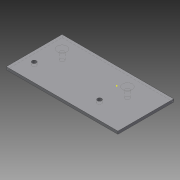
# Autodesk Inventor part: Power circuit support surface
Saved by Autodesk Inventor 2015 (Build 190159000, 159)
## iProperties
Created: 2019-05-03
Part Number: Power circuit support surface
Material: Generic
Document SubType Name: Modeling
Designer: Toby
Density: 1 g/cm^3
Appearance: Default
Author: Toby
Autodesk Inventor part; units mm, degrees
ref_plane "YZ Plane" through (0, 0, 0) normal (1, 0, 0) x (0, 1, 0)
ref_plane "XZ Plane" through (0, 0, 0) normal (0, 1, 0) x (-1, 0, 0)
ref_plane "XY Plane" through (0, 0, 0) normal (0, 0, 1) x (1, 0, 0)
sketch "Sketch1" plane through (0, 0, 0) normal (0, 0, 1) x (1, 0, 0)
  line L0 (-51.5762, 12.5065) -> (28.4238, 12.5065)
  line L1 (28.4238, 12.5065) -> (28.4238, -27.4935)
  line L2 (28.4238, -27.4935) -> (-51.5762, -27.4935)
  line L3 (-51.5762, -27.4935) -> (-51.5762, 12.5065)
  point P0 (0, 0)
  dimension "d0" = 80
  dimension "d1" = 40
  constraints: 8 end point, 2 parallel, 1 horizontal, 1 perpendicular
  measures "d0" distance between parallel lines of L1 L3
  measures "d1" distance of L2.end L0.start
extrude "Extrusion1" add sketch "Sketch1" along normal blind 2
sketch "Sketch2" plane through (0, 0, 2) normal (0, 0, 1) x (1, 0, 0)
  line L0 (-51.5762, 12.5065) -> (-51.5762, -27.4935) projected
  line L1 (-51.5762, -27.4935) -> (28.4238, -27.4935) projected
  point P0 (0, 0)
  point P1 (-44.5762, -14.4935)
  point P2 (2.2739, -14.4935)
  dimension "d4" = 46.8502
  dimension "d5" = 7
  dimension "d6" = 13
  dimension "d7" = 13
  measures "d4" distance of point (2.274, -14.494) point (-44.576, -14.494)
  measures "d5" distance from line of L0 point (-44.576, -14.494)
  measures "d6" distance from line of L1 point (-44.576, -14.494)
  measures "d7" distance from line of L1 point (2.274, -14.494)
hole "Hole1" at (-44.5762, -14.4935, 2) at (2.2739, -14.4935, 2) direction (0, 0, -1) diameter 3 depth 8 tip angle 118
sketch "Sketch3" plane through (0, 0, 2) normal (0, 0, 1) x (1, 0, 0)
  point P0 (0, 0)
sketch "Sketch4" plane through (0, 0, 0) normal (0, 0, -1) x (-1, 0, 0)
  circle A0 centre (-2.2739, -14.4935) radius 1.5 projected
  circle A1 centre (44.5762, -14.4935) radius 1.5 projected
  circle A2 centre (-2.2739, 5.5065) radius 1.5
  circle A3 centre (44.5762, 5.5065) radius 1.5
  point P0 (0, 0)
  dimension "d15" = 20
  dimension "d16" = 20
  dimension "d17" = 3
  dimension "d18" = 3
  constraints: 2 centre point, 2 coincident
  measures "d15" distance of A0.centre point (-2.274, 5.506)
  measures "d16" distance of A1.centre point (44.576, 5.506)
  measures "d17" diameter of A2
  measures "d18" diameter of A3
extrude "Extrusion2" add sketch "Sketch4" along normal blind 7 contours A2 | A3
chamfer "Chamfer1" distance 2 angle 45 2 edges at (3.7739, 5.5065, 0) (-43.0762, 5.5065, 0)
body "Solid1"
